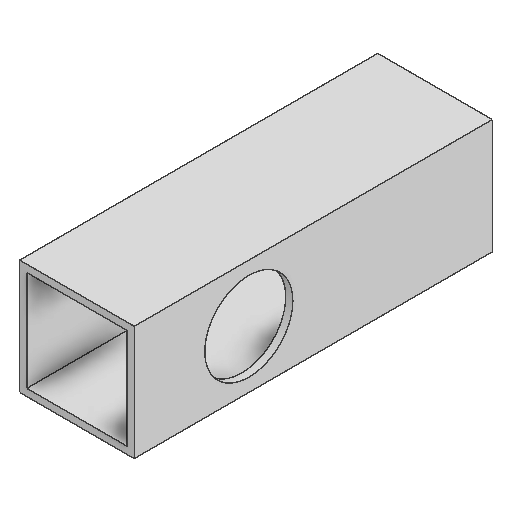
# Autodesk Inventor part: Diff Side Bar
Saved by Autodesk Inventor 2025.2 (Build 292293000, 293)
## iProperties
Created: 2025-02-20
Part Number: Diff Side Bar
Material: Generic
Document SubType Name: Modeling
Designer: Jakeg
Density: 1 g/cm^3
Appearance: Default
Author: Jakeg
Autodesk Inventor part; units mm, degrees
ref_plane "YZ Plane" through (0, 0, 0) normal (1, 0, 0) x (0, 1, 0)
ref_plane "XZ Plane" through (0, 0, 0) normal (0, 1, 0) x (-1, 0, 0)
ref_plane "XY Plane" through (0, 0, 0) normal (0, 0, 1) x (1, 0, 0)
sketch "Sketch1" plane through (0, 0, 0) normal (0, 0, 1) x (1, 0, 0)
  line L0 (-11.051, 11.5151) -> (11.174, 11.5151)
  line L1 (11.174, 11.5151) -> (11.174, -10.7099)
  line L2 (11.174, -10.7099) -> (-11.051, -10.7099)
  line L3 (-11.051, -10.7099) -> (-11.051, 11.5151)
  line L4 (-12.6385, 13.1026) -> (12.7615, 13.1026)
  line L5 (12.7615, 13.1026) -> (12.7615, -12.2974)
  line L6 (12.7615, -12.2974) -> (-12.6385, -12.2974)
  line L7 (-12.6385, -12.2974) -> (-12.6385, 13.1026)
  point P0 (0, 0)
  dimension "d0" = 25.4
  dimension "d1" = 25.4
  dimension "d2" = 1.5875
  dimension "d3" = 1.5875
  dimension "d4" = 1.5875
  dimension "d5" = 1.5875
  constraints: 16 end point, 4 parallel, 2 horizontal, 2 perpendicular
  measures "d0" distance of L4.end L5.end
  measures "d1" distance of L5.end L6.end
  measures "d2" distance between parallel lines of L6 L2
  measures "d3" distance between parallel lines of L4 L0
  measures "d4" distance between parallel lines of L7 L3
  measures "d5" distance between parallel lines of L5 L1
extrude "Extrusion1" add sketch "Sketch1" along normal blind 79.375
sketch "Sketch2" plane through (12.7615, -12.2974, 0) normal (1, 0, 0) x (0, 0, -1)
  circle A0 centre (-53.975, 12.7) radius 9.7536
  line L0 (0, 0) -> (-79.375, 0) projected
  line L1 (-79.375, 0) -> (-79.375, 25.4) projected
  circle A1 centre (-33.655, 12.7) radius 3.175
  circle A2 centre (-74.295, 12.7) radius 3.175
  point P0 (0, 12.2974)
  dimension "d8" = 19.5072
  dimension "d11" = 12.7
  dimension "d12" = 25.4
  dimension "d13" = 20.32
  dimension "d14" = 6.35
  dimension "d15" = 6.35
  dimension "d16" = 20.32
  constraints: 3 centre point
  measures "d8" diameter of A0
  measures "d11" distance from line of L0 A0.centre
  measures "d12" distance from line of L1 A0.centre
  measures "d13" distance of A1.centre A0.centre
  measures "d14" diameter of A1
  measures "d15" diameter of A2
  measures "d16" distance of A0.centre A2.centre
extrude "Extrusion2" cut sketch "Sketch2" against normal through all contours A0
equation "\"d3\" = d2"
equation "\"d4\" = d2"
equation "\"d5\" = d2"
equation "\"d16\" = d13"
body "Solid1"
